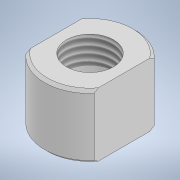
# Autodesk Inventor part: Port Conversion Nut
Saved by Autodesk Inventor 2021 (Build 250183000, 183)
## iProperties
Created: 2020-07-21
Part Number: Port Conversion Nut
Material: Generic
Document SubType Name: Modeling
Designer: jgray
Density: 1 g/cm^3
Appearance: Default
Author: jgray
Autodesk Inventor part; units mm, degrees
ref_plane "YZ Plane" through (0, 0, 0) normal (1, 0, 0) x (0, 1, 0)
ref_plane "XZ Plane" through (0, 0, 0) normal (0, 1, 0) x (-1, 0, 0)
ref_plane "XY Plane" through (0, 0, 0) normal (0, 0, 1) x (1, 0, 0)
sketch "Sketch1" plane through (0, 0, 0) normal (0, 1, 0) x (-1, 0, 0)
  circle A0 centre (0, 0) radius 10
  dimension "d0" = 20
  constraints: 1 centre point, 1 coincident
  measures "d0" diameter of A0
extrude "Extrusion1" add sketch "Sketch1" along normal blind 14
sketch "Sketch2" plane through (0, 14, 0) normal (0, 1, 0) x (1, 0, 0)
  point P0 (0, 0)
  point P1 (0, 0)
  constraints: 1 coincident
hole "Hole1" at (0, 14, 0) direction (0, -1, 0) diameter 10.376 depth 9 tip angle 118 thread size "M12x1.5" class "6H" standard "ISO Metric profile"
sketch "Sketch3" plane through (0, 0, 0) normal (0, -1, 0) x (1, 0, 0)
  point P0 (0, 0)
  point P1 (0, 0)
  constraints: 1 coincident
hole "Hole2" at (0, 0, 0) direction (0, 1, 0) diameter 3.9624 end through all thread size "10-32 UNF" class "2B" standard "ANSI Unified Screw Threads"
chamfer "Chamfer1" distance 0.6 angle 45 3 edges at (0, 0, 1.9812) (10, 14, 0) (10, 0, 0)
sketch "Sketch4" plane through (0, 0, 0) normal (0, -1, 0) x (1, 0, 0)
  circle A0 centre (0, 0) radius 5.188 projected
  circle A1 centre (0, 0) radius 10 projected
  line L0 (-7.5, 6.6144) -> (7.5, 6.6144)
  line L1 (7.5, 6.6144) -> (7.5, -6.6144)
  line L2 (7.5, -6.6144) -> (-7.5, -6.6144)
  line L3 (-7.5, -6.6144) -> (-7.5, 6.6144)
  circle A2 centre (0, 0) radius 2.5812 projected
  line L4 (-7.5, 6.6144) -> (7.5, -6.6144) construction
  line L5 (7.5, 6.6144) -> (-7.5, -6.6144) construction
  point P0 (-7.5, -6.6144)
  point P1 (-7.5, 6.6144)
  point P2 (7.5, 6.6144)
  dimension "d20" = 15
  constraints: 12 end point, 2 midpoint, 2 parallel, 1 horizontal, 1 perpendicular, 2 other
  measures "d20" distance of L1.end L2.end
extrude "Extrusion2" cut sketch "Sketch4" against normal blind 14 contours A1 L1 | L3 A1
body "Solid1"
